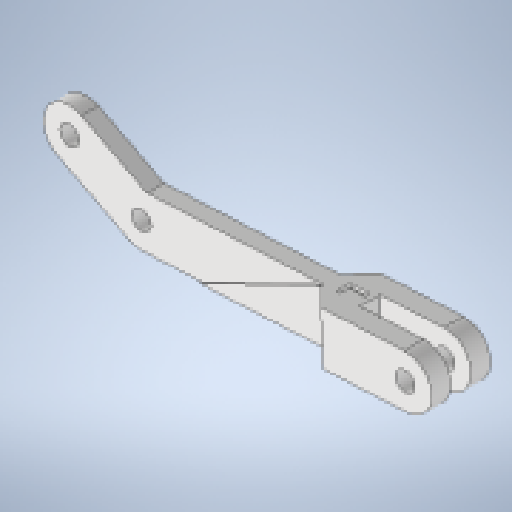
# Autodesk Inventor part: GripperShaftLeft
Saved by Autodesk Inventor 2025.1 (Build 291241000, 241)
## iProperties
Created: 2026-05-06
Part Number: GripperShaftLeft
Material: Generic
Document SubType Name: Modeling
Designer: User
Density: 1 g/cm^3
Appearance: Default
Author: User
## iProperties of the stored document GripperShaftLeft_3DPrint.ipt
Created: 2026-05-06
Part Number: GripperShaftLeft_3DPrint
Material: Generic
Document SubType Name: Modeling
Designer: User
Density: 1 g/cm^3
Appearance: Default
Author: User
Autodesk Inventor part; units mm, degrees
ref_plane "YZ Plane" through (0, 0, 0) normal (1, 0, 0) x (0, 1, 0)
ref_plane "XZ Plane" through (0, 0, 0) normal (0, 1, 0) x (-1, 0, 0)
ref_plane "XY Plane" through (0, 0, 0) normal (0, 0, 1) x (1, 0, 0)
sketch "Sketch1" plane through (0, 0, 0) normal (0, 0, 1) x (1, 0, 0)
  line L0 (-26.2933, 15.2055) -> (-26.6969, 23.1953) projected
  line L1 (-26.6969, 23.1953) -> (-13.9216, 23.8407) projected
  arc A0 (-13.518, 15.8509) -> (-13.9216, 23.8407) centre (-13.7198, 19.8458) ccw projected
  line L2 (-13.518, 15.8509) -> (-26.2933, 15.2055) projected
  circle A1 centre (-13.7198, 19.8458) radius 1.5 projected
  point P0 (0, 0)
extrude "Extrusion1" add sketch "Sketch1" along normal blind 3
sketch "Sketch2" plane through (0, 0, 0) normal (0, 0, -1) x (-1, 0, 0)
  line L0 (23.7008, 23.3467) -> (23.2971, 15.3569) projected
  line L1 (26.6969, 23.1953) -> (26.2933, 15.2055) projected
  line L2 (13.9216, 23.8407) -> (26.6969, 23.1953) projected
  arc A0 (13.9216, 23.8407) -> (13.518, 15.8509) centre (13.7198, 19.8458) ccw projected
  line L3 (26.2933, 15.2055) -> (13.518, 15.8509) projected
  line L4 (26.6969, 23.1953) -> (26.2933, 15.2055) projected
  circle A1 centre (13.7198, 19.8458) radius 1.5 projected
  point P0 (0, 0)
extrude "Extrusion2" add sketch "Sketch2" along normal blind 3.1 contours L2 L1 L3 L0
sketch "Sketch3" plane through (0, 0, -3.1) normal (0, 0, -1) x (-1, 0, 0)
  line L0 (13.9216, 23.8407) -> (26.6969, 23.1953) projected
  line L1 (26.6969, 23.1953) -> (26.2933, 15.2055) projected
  line L2 (26.2933, 15.2055) -> (13.518, 15.8509) projected
  arc A0 (13.9216, 23.8407) -> (13.518, 15.8509) centre (13.7198, 19.8458) ccw projected
  circle A1 centre (13.7198, 19.8458) radius 1.5 projected
  point P0 (0, 0)
extrude "Extrusion3" add sketch "Sketch3" along normal blind 3
sketch "Sketch4" plane through (0, 0, 0) normal (0, 0, -1) x (-1, 0, 0)
  arc A0 (57.4536, 13.6314) -> (57.8572, 21.6212) centre (57.6554, 17.6263) ccw projected
  line L0 (57.4536, 13.6314) -> (29.3894, 15.0491) projected
  line L1 (29.793, 23.0389) -> (29.3894, 15.0491) projected
  line L2 (29.793, 23.0389) -> (57.8572, 21.6212) projected
  circle A1 centre (57.6554, 17.6263) radius 1.5 projected
  line L3 (29.3894, 15.0491) -> (26.2933, 15.2055) projected
  line L4 (26.6969, 23.1953) -> (26.2933, 15.2055) projected
  line L5 (26.6969, 23.1953) -> (29.793, 23.0389) projected
  line L6 (29.793, 23.0389) -> (29.3894, 15.0491) projected
  circle A2 centre (68.6887, 23.3886) radius 1.5 projected
  arc A3 (70.5404, 19.843) -> (66.837, 26.9342) centre (68.6887, 23.3886) ccw
  line L7 (59.5071, 14.0807) -> (70.5404, 19.843)
  arc A4 (57.4536, 13.6314) -> (57.8572, 21.6212) centre (57.6554, 17.6263) ccw
  line L8 (56.7692, 21.6761) -> (66.837, 26.9342)
  point P0 (0, 0)
  dimension "d18" = 8
  constraints: 6 end point, 5 point on circle, 4 tangent, 2 centre point, 2 coincident, 1 concentric, 1 point on line
  measures "d18" diameter of A3
extrude "Extrusion4" add sketch "Sketch4" along normal blind 3
chamfer "Chamfer1" distance 3 angle 45 1 edges at (-26.4951, 19.2004, 0)
chamfer "Chamfer2" distance 3.1 angle 45 1 edges at (-26.4951, 19.2004, -3)
ref_plane "Work Plane1" through (-62.9426, 1.3124, -0.3887) normal (0, 0, -1) x (-0.0504539, 0.9987264, 0)
sketch "Sketch6" plane through (0, 0, 0) normal (0, 0, 1) x (1, 0, 0)
  line L0 (-57.4536, 13.6314) -> (-48.2653, 14.0955) projected
  arc A0 (-57.8572, 21.6212) -> (-57.4536, 13.6314) centre (-57.6554, 17.6263) ccw projected
  line L1 (-29.6931, 23.044) -> (-57.8572, 21.6212) projected
  line L2 (-29.6931, 23.044) -> (-48.2653, 14.0955) projected
  circle A1 centre (-57.6554, 17.6263) radius 1.5 projected
  point P0 (0, 0)
extrude "Extrusion5" cut sketch "Sketch6" against normal up to surface (0.3887 mm away)
sketch "Sketch7" plane through (-13.9216, 23.8407, 3) normal (-0.0504539, 0.9987264, 0) x (0.9987264, 0.0504539, 0)
  line L0 (-10.7481, 5.8068) -> (-10.7481, 3.4068) construction
  line L1 (-10.7481, 3.4068) -> (-13.7981, 3.4068) construction
  line L2 (-13.7981, 3.4068) -> (-13.7981, 5.8068) construction
  line L3 (-13.7981, 5.8068) -> (-10.7481, 5.8068) construction
  line L4 (-13.7981, 3.4562) -> (-13.7981, 5.4904)
  line L5 (-13.7981, 5.4904) -> (-10.7481, 5.4904)
  line L6 (-10.7481, 5.4904) -> (-10.7481, 4.7242)
  line L7 (-10.7481, 4.7242) -> (-13.2172, 4.7242)
  line L8 (-13.2172, 4.7242) -> (-13.2172, 3.4562)
  line L9 (-13.2172, 3.4562) -> (-13.7981, 3.4562)
  point P0 (12.701, 3)
  constraints: 2 other
emboss "Emboss1" sketch "Sketch7" operation cut depth 0.5 direction (0.0504539, -0.9987264, 0)
sketch "Sketch8" plane through (0, 0, 0) normal (0, 0, 1) x (1, 0, 0)
  line L0 (-57.8572, 21.6212) -> (-56.7692, 21.6761) projected
  line L1 (-66.837, 26.9342) -> (-56.7692, 21.6761) projected
  arc A0 (-66.837, 26.9342) -> (-70.5404, 19.843) centre (-68.6887, 23.3886) ccw projected
  line L2 (-59.5071, 14.0807) -> (-70.5404, 19.843) projected
  arc A1 (-57.8572, 21.6212) -> (-59.5071, 14.0807) centre (-57.6554, 17.6263) ccw projected
  circle A2 centre (-68.6887, 23.3886) radius 1.5 projected
  point P0 (0, 0)
extrude "Extrusion6" cut sketch "Sketch8" against normal up to surface (0.3887 mm away)
body "Solid1"
